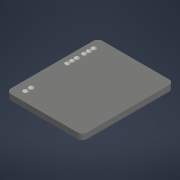
# Autodesk Inventor part: Tapa Case
Saved by Autodesk Inventor 2021 (Build 250183000, 183)
## iProperties
Created: 2021-03-29
Part Number: Tapa Case
Material: Genérico
Document SubType Name: Modeling
Designer: grego
Density: 1 g/cm^3
Appearance: Valor por defecto
Author: grego
Autodesk Inventor part; units mm, degrees
ref_plane "YZ Plane" through (0, 0, 0) normal (1, 0, 0) x (0, 1, 0)
ref_plane "XZ Plane" through (0, 0, 0) normal (0, 1, 0) x (-1, 0, 0)
ref_plane "XY Plane" through (0, 0, 0) normal (0, 0, 1) x (1, 0, 0)
sketch "Boceto1" plane through (0, 0, 0) normal (0, 1, 0) x (-1, 0, 0)
  line L0 (-5, 0) -> (-75.1, 0)
  line L1 (-80.1, -5) -> (-80.1, -91.5)
  line L2 (-75.1, -96.5) -> (-5, -96.5)
  line L3 (0, -91.5) -> (0, -5)
  arc A0 (0, -5) -> (-5, 0) centre (-5, -5) ccw
  arc A1 (-75.1, 0) -> (-80.1, -5) centre (-75.1, -5) ccw
  arc A2 (-80.1, -91.5) -> (-75.1, -96.5) centre (-75.1, -91.5) ccw
  arc A3 (-5, -96.5) -> (0, -91.5) centre (-5, -91.5) ccw
  point P0 (0, 0)
  point P1 (-80.1, -96.5)
  point P2 (-80.1, 0)
  point P3 (0, -96.5)
  dimension "d0" = 96.5
  dimension "d1" = 80.1
  dimension "d2" = 5
  constraints: 8 end point, 8 point on circle, 8 point on line, 8 tangent, 4 centre point, 3 equal radius, 2 parallel, 1 horizontal, 1 perpendicular
  measures "d0" distance of point (-80.1, 0) point (-80.1, -96.5)
  measures "d1" distance of point (-80.1, -96.5) point (0, -96.5)
  measures "d2" radius of A0
extrude "Extrusión1" add sketch "Boceto1" along normal blind 6
sketch "Boceto2" plane through (0, 0, 0) normal (0, -1, 0) x (1, 0, 0)
  circle A0 centre (10.2, -10.54) radius 2.5
  circle A1 centre (10.2, -16.54) radius 2.5
  circle A2 centre (7.06, -57.64) radius 2.4
  circle A3 centre (7.06, -62.64) radius 2.4
  circle A4 centre (7.06, -67.64) radius 2.4
  circle A5 centre (7.08, -75.21) radius 2.4
  circle A6 centre (7.08, -80.21) radius 2.4
  circle A7 centre (7.08, -85.21) radius 2.4
  point P0 (0, 0)
  constraints: 8 centre point
extrude "Extrusión2" cut sketch "Boceto2" against normal blind 10
sketch "Boceto3" plane through (0, 6, 0) normal (0, 1, 0) x (1, 0, 0)
  line L0 (6.9461, 7.6948) -> (13.2683, 7.6948)
  line L1 (13.2683, 7.6948) -> (13.2683, 19.5905)
  line L2 (13.2683, 19.5905) -> (6.9461, 19.5905)
  line L3 (6.9461, 19.5905) -> (6.9461, 7.6948)
  circle A0 centre (10.2, 16.54) radius 2.5 projected
  circle A1 centre (10.2, 10.54) radius 2.5 projected
  point P0 (0, 0)
  constraints: 8 end point, 2 parallel, 1 horizontal, 1 perpendicular
extrude "Extrusión3" add sketch "Boceto3" along normal blind 15
fillet "Empalme1" radius 3 4 edges at (6.9461, 13.5, -19.5905) (6.9461, 13.5, -7.6948) (13.2683, 13.5, -7.6948) (13.2683, 13.5, -19.5905)
sketch "Boceto4" plane through (0, 6, 0) normal (0, 1, 0) x (1, 0, 0)
  line L0 (3.9852, 54.3304) -> (10.0586, 54.3304)
  line L1 (10.0586, 54.3304) -> (10.0586, 88.8384)
  line L2 (10.0586, 88.8384) -> (3.9852, 88.8384)
  line L3 (3.9852, 88.8384) -> (3.9852, 54.3304)
  circle A0 centre (7.06, 57.64) radius 2.4 projected
  circle A1 centre (7.06, 62.64) radius 2.4 projected
  circle A2 centre (7.06, 67.64) radius 2.4 projected
  circle A3 centre (7.08, 75.21) radius 2.4 projected
  circle A4 centre (7.08, 80.21) radius 2.4 projected
  circle A5 centre (7.08, 85.21) radius 2.4 projected
  point P0 (0, 0)
  constraints: 8 end point, 2 parallel, 1 horizontal, 1 perpendicular
extrude "Extrusión4" add sketch "Boceto4" along normal blind 15
fillet "Empalme2" radius 3 4 edges at (3.9852, 13.5, -54.3304) (3.9852, 13.5, -88.8384) (10.0586, 13.5, -88.8384) (10.0586, 13.5, -54.3304)
